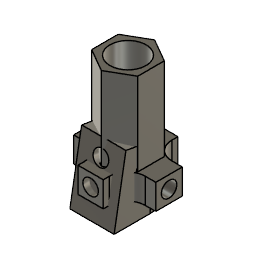
Steering absolute encoder (Autodesk Fusion 360 design; units mm, degrees)
Autodesk Fusion 360 part; units mm, degrees
sketch "Skizze1" plane through (0, 0, 0) normal (0, 0, 1) x (1, 0, 0)
  circle A0 centre (0, 0) radius 5
  line L0 (6.4, 3.695) -> (0, 7.3901)
  line L1 (0, 7.3901) -> (-6.4, 3.695)
  line L2 (-6.4, 3.695) -> (-6.4, -3.695)
  line L3 (-6.4, -3.695) -> (0, -7.3901)
  line L4 (0, -7.3901) -> (6.4, -3.695)
  line L5 (6.4, -3.695) -> (6.4, 3.695)
  dimension "d1" = 10
  dimension "d2" = 12.8
  constraint coincident A0.centre origin
  constraint vertical L5
  measures "d1" diameter of A0
  measures "d2" distance of L2 L5
extrude "Extrusion1" add sketch "Skizze1" along normal blind 30 makes body 1
ref_plane "Arbeitsebene1" through (12.125, 0, 0) normal (0, 0.984808, -0.173648) x (1, 0, 0)
sketch "Skizze2" plane through (0, 0, 0) normal (0, 0, 1) x (1, 0, 0)
  circle A0 centre (0, 0) radius 2.15
  circle A1 centre (0, 0) radius 6.15
  circle A2 centre (0, 0) radius 4
  line L0 (6.15, 0) -> (6.15, -10)
  line L1 (6.15, -10) -> (-6.15, -10)
  line L2 (-6.15, -10) -> (-6.15, 0)
  dimension "d6" = 4.3
  dimension "d7" = 4
  dimension "d8" = 8
  dimension "d9" = 10
  constraint coincident A0.centre A1.centre
  constraint coincident A1 L0.start
  constraint tangent A1 L0
  constraint vertical L0
  constraint perpendicular L0 L1
  constraint coincident A1 L2.end
  constraint tangent A1 L2
  constraint vertical L2
  measures "d6" diameter of A0
  measures "d7" distance of A0 A1
  measures "d8" diameter of A2
  measures "d9" distance of L1.end L2.end
extrude "Extrusion2" add sketch "Skizze2" against normal blind 5 separate body contours A1 | A1 L0 L1 L2 | A2 makes body 2
extrude "Extrusion3" add sketch "Skizze2" along normal blind 3 contours A1 | A1 L0 L1 L2 bodies 2
sketch "Skizze3" plane through (6.15, 0, 0) normal (1, 0, 0) x (0, 1, 0)
  line L0 (-10, 3) -> (-10, -5)
  line L1 (-10, -5) -> (0, -5)
  line L2 (0, -5) -> (0, 3)
  line L3 (0, 3) -> (-10, 3)
  line L4 (-4, 3) -> (4, 3)
  line L5 (4, 0) -> (-4, 0)
  line L6 (-10, -5) -> (-6.7304, 13.5427)
  line L7 (-6.7304, 13.5427) -> (-2.7912, 12.8481)
  line L8 (-2.7912, 12.8481) -> (-4.5277, 3)
  line L9 (0, 0) -> (-3.5, 0) construction
  line L10 (-3.5, 0) -> (-3.5, 11.5029) construction
  line L11 (-7.1385, 11.2284) -> (-3.1993, 10.5338) construction
  line L12 (-7.8852, 6.9937) -> (-3.946, 6.2991) construction
  line L13 (-3.946, 6.2991) -> (14.7642, 3) construction
  line L14 (-6.9041, 12.5579) -> (-2.9648, 11.8633) construction
  line L15 (-8.1196, 5.6642) -> (-4.1804, 4.9696) construction
  line L16 (-7.2671, 5.5139) -> (-7.0327, 6.8434) construction
  line L17 (-6.1742, 11.0583) -> (-5.9398, 12.3878) construction
  line L18 (0, 3) -> (0, -5)
  line L19 (0, -5) -> (6.15, -5)
  line L20 (0, -5) -> (0, 3)
  line L21 (6.15, 3) -> (0, 3)
  dimension "d14" = 10
  dimension "d15" = 4
  dimension "d16" = 3.5
  dimension "d17" = 4.3
  dimension "d18" = 7
  dimension "d19" = 1
  dimension "d31" = 2
  constraint coincident L0.end L1.start
  constraint perpendicular L6 L7
  constraint coincident L3 L8.end
  constraint perpendicular L7 L8
  constraint coincident L9.start origin
  constraint perpendicular L2 L9
  constraint coincident L6 L11.start
  constraint coincident L8 L11.end
  constraint perpendicular L8 L11
  constraint coincident L6 L12.start
  constraint coincident L8 L12.end
  constraint perpendicular L8 L12
  constraint parallel L12 L13
  constraint coincident L6 L14.start
  constraint coincident L8 L14.end
  constraint perpendicular L8 L14
  constraint coincident L6 L15.start
  constraint perpendicular L8 L15
  constraint coincident L15 L16.start
  constraint coincident L12 L16.end
  constraint perpendicular L12 L16
  constraint coincident L11 L17.start
  constraint coincident L14 L17.end
  constraint perpendicular L14 L17
  constraint equal L16 L17
  constraint vertical L10
  constraint horizontal L4.end L13.end
  constraint coincident L8 L15.end
  measures "d14" angle of L0 L6
  measures "d15" distance of L6.end L7.end
  measures "d16" distance of L9.start L9.end
  measures "d17" distance of L11 L12
  measures "d18" distance of L14 L15
  measures "d19" distance of L7 L14
  measures "d31" distance of L8.end L15.end
extrude "Extrusion4" cut sketch "Skizze3" against normal through all contours L0 L3 L6 bodies 2
extrude "Extrusion5" add sketch "Skizze3" against normal up to surface (12.3 mm away) contours L3 L6 L7 L8 bodies 2
fillet "Abrundung1" radius 2.5 1 edges at (0, -4.5277, 3) on bodies 2
sketch "Skizze4" plane through (0, -8.8434, 1.5593) normal (0, -0.984808, 0.173648) x (1, 0, 0)
  line L0 (-6.15, 12.1682) -> (-6.15, -6.6605)
  line L1 (-6.15, -6.6605) -> (6.15, -6.6605)
  line L2 (6.15, -6.6605) -> (6.15, 12.1682)
  line L3 (6.15, 12.1682) -> (-6.15, 12.1682)
  line L4 (6.15, 9.8182) -> (6.15, 5.5182) construction
  line L5 (6.15, 7.6682) -> (-6.15, 7.6682) construction
  circle A0 centre (0, 7.6682) radius 2.15
  line L6 (2.0207, 11.1682) -> (-2.0207, 11.1682)
  line L7 (-2.0207, 11.1682) -> (-4.0415, 7.6682)
  line L8 (-4.0415, 7.6682) -> (-2.0207, 4.1682)
  line L9 (-2.0207, 4.1682) -> (2.0207, 4.1682)
  line L10 (2.0207, 4.1682) -> (4.0415, 7.6682)
  line L11 (4.0415, 7.6682) -> (2.0207, 11.1682)
  point P0 (6.15, 9.8182)
  point P1 (6.15, 5.5182)
  point P2 (0, 7.6682)
  dimension "d25" = 4.3
  dimension "d26" = 7
  constraint coincident P0 L4.start
  constraint coincident P1 L4.end
  constraint midpoint L4 L5.start
  constraint coincident L0 L5.end
  constraint perpendicular L0 L5
  constraint midpoint L5 P2
  constraint coincident P2 A0.centre
  constraint horizontal L6
  measures "d25" diameter of A0
  measures "d26" distance of L6 L9
extrude "Extrusion6" cut sketch "Skizze4" against normal through all contours A0 bodies 2
extrude "Extrusion7" cut sketch "Skizze4" against normal through all from surface at -2 contours L6 L7 L8 L9 L10 L11 bodies 2
sketch "Skizze5" plane through (0, 0, 0) normal (0, 0, 1) x (1, 0, 0)
  circle A0 centre (0, 0) radius 5
  line L0 (6.4, 3.695) -> (6.4, -3.695)
  line L1 (6.4, -3.695) -> (0, -7.3901)
  line L2 (0, -7.3901) -> (-6.4, -3.695)
  line L3 (-6.4, -3.695) -> (-6.4, 3.695)
  line L4 (-6.4, 3.695) -> (0, 7.3901)
  line L5 (0, 7.3901) -> (6.4, 3.695)
  line L6 (-3.5, -5.3694) -> (3.5, -5.3694)
  line L7 (3.5, -5.3694) -> (3.5, -10.3694)
  line L8 (3.5, -10.3694) -> (-3.5, -10.3694)
  line L9 (-3.5, -10.3694) -> (-3.5, -5.3694)
  line L10 (6.4, 3.695) -> (11.4, 3.695)
  line L11 (11.4, 3.695) -> (11.4, -3.695)
  line L12 (11.4, -3.695) -> (6.4, -3.695)
  line L13 (6.4, -3.695) -> (6.4, 3.695)
  line L14 (20, 0) -> (2.5, 0)
  line L15 (3.5, 10.3694) -> (-3.5, 10.3694)
  line L16 (3.5, 5.3694) -> (3.5, 10.3694)
  line L17 (-3.5, 10.3694) -> (-3.5, 5.3694)
  line L18 (0, 2.5) -> (0, 20)
  line L19 (-11.4, -3.695) -> (-6.4, -3.695)
  line L20 (-11.4, 3.695) -> (-11.4, -3.695)
  line L21 (-6.4, 3.695) -> (-11.4, 3.695)
  point P0 (0, -5.3694)
  point P1 (6.4, 0)
  dimension "d32" = 7
  dimension "d34" = 5
  dimension "d35" = 5
  constraint horizontal L6
  constraint vertical L7
  constraint horizontal L8
  constraint vertical L9
  constraint coincident L2 L6.start
  constraint horizontal L10
  constraint vertical L11
  constraint horizontal L12
  constraint vertical L13
  constraint coincident L0 L5.end
  constraint midpoint L6 P0
  constraint midpoint L13 P1
  constraint vertical A0.centre P0
  constraint horizontal A0.centre P1
  constraint symmetric L6.start L14 L17.end
  constraint symmetric L6.end L14 L16.start
  constraint symmetric L7.end L14 L15.start
  constraint symmetric L8.end L14 L15.end
  constraint symmetric L0.start L18 L3.end
  constraint symmetric L10.end L18 L20.start
  constraint symmetric L11.end L18 L19.start
  constraint symmetric L0.end L18 L2.end
  constraint coincident L0.end L1.start
  measures "d32" distance of L7.end L8.end
  measures "d34" distance of L6.end L7.end
  measures "d35" distance of L11.end L0.end
extrude "Extrusion8" add sketch "Skizze5" along normal blind 7 contours L0 L11 L12 L13 L14 | L0 L10 L11 L13 L14 | L5 L15 L16 L18 | L4 L15 L17 L18 | L1 L2 L7 L8 L9 | L3 L19 L20 L21 bodies 1
split "Teilen1" by plane through (0, 0, 7) normal (0, 0, 1) bodies 1 makes body 3 at (4.9752, 0.4978, 14.6667)
fillet "Abrundung2" radius 5 8 edges at (-6.4, -3.695, 3.5) (-3.5, -5.3694, 3.5) (-6.4, 3.695, 3.5) (-3.5, 5.3694, 3.5) (3.5, 5.3694, 3.5) (6.4, 3.695, 3.5) (6.4, -3.695, 3.5) (3.5, -5.3694, 3.5) on bodies 1
combine "Kombinieren1" operation add target body 3 tool bodies 1
sketch "Skizze6" plane through (0, -10.3694, 0) normal (0, -1, 0) x (1, 0, 0)
  line L0 (-3.5, 0) -> (3.5, 0)
  line L1 (3.5, 0) -> (3.5, 7)
  line L2 (3.5, 7) -> (-3.5, 7)
  line L3 (-3.5, 7) -> (-3.5, 0)
  line L4 (0, 0) -> (0, 7) construction
  circle A0 centre (0, 3.5) radius 2.15
  dimension "d40" = 4.3
  constraint coincident L4.start origin
  constraint midpoint L2 L4.end
  constraint midpoint L4 A0.centre
  measures "d40" diameter of A0
extrude "Extrusion9" cut sketch "Skizze6" against normal through all contours A0 bodies 3
sketch "Skizze7" plane through (-11.4, 0, 0) normal (-1, 0, 0) x (0, -1, 0)
  line L0 (-3.695, 0) -> (3.695, 0)
  line L1 (3.695, 0) -> (3.695, 7)
  line L2 (3.695, 7) -> (-3.695, 7)
  line L3 (-3.695, 7) -> (-3.695, 0)
  line L4 (0, 0) -> (0, 7) construction
  circle A0 centre (0, 3.5) radius 2.15
  dimension "d42" = 4.3
  constraint coincident L4.start origin
  constraint midpoint L2 L4.end
  constraint midpoint L4 A0.centre
  measures "d42" diameter of A0
extrude "Extrusion10" cut sketch "Skizze7" against normal through all contours A0 bodies 3
